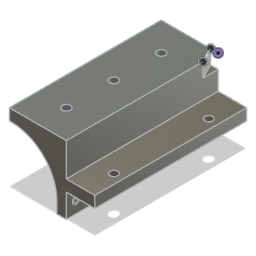
rear_mount_right_v2 (Autodesk Fusion 360 design; units mm, degrees)
Autodesk Fusion 360 part; units mm, degrees
note: some values were not read from the file. Set by a fixed rule: which sketch regions a step uses.
sketch "Esquisse1" plane through (0, 0, 0) normal (0, 0, 1) x (1, 0, 0)
  line L0 (15, 0) -> (0, 0)
  line L1 (0, 0) -> (0, 17.5)
  line L2 (0, 17.5) -> (-30, 17.5)
  line L3 (-30, 17.5) -> (-30, 11.5)
  line L4 (-30, 11.5) -> (-5, 11.5)
  line L5 (-5, 11.5) -> (-5, -18.5)
  line L6 (-5, -18.5) -> (0, -18.5)
  line L7 (0, -18.5) -> (0, -6)
  line L8 (0, -6) -> (15, -6)
  line L9 (15, -6) -> (15, 0)
  dimension "d1" = 12.5
  dimension "d2" = 6
  dimension "d3" = 5
  dimension "d4" = 15
  dimension "d6" = 6
  dimension "d7" = 30
  dimension "d46" = 36
  constraint coincident L0.end L1.start
  constraint horizontal L0
  constraint perpendicular L0 L1
  constraint perpendicular L1 L2
  constraint perpendicular L2 L3
  constraint perpendicular L3 L4
  constraint perpendicular L4 L5
  constraint perpendicular L5 L6
  constraint perpendicular L6 L7
  constraint perpendicular L7 L8
  constraint perpendicular L0 L9
  constraint collinear L1 L7
  measures "d1" distance of L6.end L7.end
  measures "d2" distance of L0.start L8.end
  measures "d3" distance of L5.end L6.end
  measures "d4" distance of L0.start L0.end
  measures "d6" distance of L2.end L3.end
  measures "d7" distance of L1 L3
  measures "d46" distance of L2 L6
extrude "Extrusion1" add sketch "Esquisse1" along normal blind 80
sketch "Esquisse2" plane through (0, -6, 0) normal (0, -1, 0) x (1, 0, 0)
  line L0 (0, 0) -> (15, 0)
  line L1 (15, 0) -> (15, 80)
  line L2 (15, 80) -> (0, 80)
  line L3 (0, 80) -> (0, 0)
  line L4 (10, 80) -> (10, 0) construction
  circle A0 centre (10, 65) radius 2.075
  circle A1 centre (10, 15) radius 2.075
  dimension "d10" = 4.15
  dimension "d11" = 15
  dimension "d12" = 15
  dimension "d38" = 10
  constraint coincident L4 A0.centre
  constraint coincident L4 A1.centre
  constraint equal A0 A1
  constraint vertical L4
  measures "d10" diameter of A1
  measures "d11" distance of L2 A0.centre
  measures "d12" distance of L0 A1.centre
  measures "d38" distance of L0.start L4
extrude "Extrusion2" cut sketch "Esquisse2" against normal blind 10 contours A0 | A1
sketch "Esquisse3" plane through (-5, 0, 0) normal (-1, 0, 0) x (0, 0, 1)
  line L0 (0, 11.5) -> (0, -18.5)
  line L1 (0, -18.5) -> (80, -18.5)
  line L2 (80, -18.5) -> (80, 11.5)
  line L3 (80, 11.5) -> (0, 11.5)
  line L4 (80, -12.25) -> (-7.1825, -12.25) construction
  circle A0 centre (19.5, -12.25) radius 1.75
  circle A1 centre (68, -12.25) radius 1.75
  circle A2 centre (75, -12.25) radius 1.75
  dimension "d15" = 6.25
  dimension "d16" = 3.5
  dimension "d17" = 5
  dimension "d18" = 7
  dimension "d19" = 60.5
  constraint coincident L2 L4.start
  constraint perpendicular L0 L4
  constraint coincident L4 A0.centre
  constraint coincident L4 A1.centre
  constraint coincident L4 A2.centre
  constraint equal A0 A1
  constraint equal A1 A2
  measures "d15" distance of L1 L4
  measures "d16" diameter of A0
  measures "d17" distance of L2 A2.centre
  measures "d18" distance of A1.centre A2.centre
  measures "d19" distance of L2 A0.centre
extrude "Extrusion3" cut sketch "Esquisse3" against normal blind 5 contours A0 | A1 | A2
fillet "Congé1" radius 24 1 edges at (-5, 11.5, 40)
sketch "Esquisse4" plane through (0, 17.5, 0) normal (0, 1, 0) x (-1, 0, 0)
  line L0 (0, 0) -> (30, 0)
  line L1 (30, 0) -> (30, 80)
  line L2 (30, 80) -> (0, 80)
  line L3 (0, 80) -> (0, 0)
  line L4 (15, 0) -> (15, 80) construction
  circle A0 centre (15, 15) radius 2.175
  circle A1 centre (15, 40) radius 2.175
  circle A2 centre (15, 65) radius 2.175
  dimension "d25" = 4.35
  dimension "d26" = 40
  dimension "d27" = 15
  dimension "d28" = 15
  dimension "d36" = 65
  dimension "d37" = 15
  dimension "d44" = 15
  constraint coincident L0 L4.start
  constraint perpendicular L2 L4
  constraint coincident L4 A0.centre
  constraint midpoint L4 A1.centre
  constraint coincident L4 A2.centre
  constraint equal A1 A2
  constraint equal A0 A1
  measures "d25" diameter of A2
  measures "d26" distance of L2 A1.centre
  measures "d27" distance of L2 A2.centre
  measures "d28" distance of L0 A0.centre
  measures "d36" distance of L4.end A0.centre
  measures "d37" distance of L2.end L4.end
  measures "d44" distance of L1.end L4.end
extrude "Extrusion4" cut sketch "Esquisse4" against normal blind 33 contours A0 | A1 | A2
sketch "Esquisse5" plane through (0, 17.5, 0) normal (0, 1, 0) x (-1, 0, 0)
  circle A0 centre (15, 15) radius 2.175
  circle A1 centre (15, 40) radius 2.175
  circle A2 centre (15, 65) radius 2.175
  line L0 (0, 0) -> (30, 0)
  line L1 (30, 0) -> (30, 80)
  line L2 (30, 80) -> (0, 80)
  line L3 (0, 80) -> (0, 0)
  line L4 (0, 8) -> (4, 0)
  dimension "d31" = 8
  dimension "d32" = 4
  constraint coincident L3 L4.start
  constraint coincident L0 L4.end
  measures "d31" distance of L0.start L4.start
  measures "d32" distance of L0.start L4.end
extrude "Extrusion5" cut sketch "Esquisse5" against normal blind 7.5 contours L0 L3 L4
sketch "Esquisse6" plane through (0, 11.5, 0) normal (0, -1, 0) x (1, 0, 0)
  line L0 (-29, 0) -> (-29, 80)
  line L1 (-29, 80) -> (-30, 80)
  line L2 (-30, 80) -> (-30, 0)
  line L3 (-30, 0) -> (-29, 0)
  circle A0 centre (-15, 15) radius 4
  circle A1 centre (-15, 40) radius 4
  circle A2 centre (-15, 65) radius 4
  dimension "d39" = 8
  constraint equal A1 A2
  constraint equal A0 A1
  measures "d39" diameter of A1
extrude "Extrusion6" cut sketch "Esquisse6" along normal blind 16 contours A0 | A1 | A2
sketch "Esquisse8" plane through (0, 12.5, 0) normal (0, -1, 0) x (1, 0, 0)
  circle A0 centre (-15, 65) radius 1.575
  circle A1 centre (-15, 65) radius 2.175
  circle A2 centre (-15, 65) radius 4
  circle A3 centre (-15, 14.9898) radius 4
  circle A4 centre (-15, 40) radius 4
  circle A5 centre (-15, 40) radius 2.175
  dimension "d45" = 8
  constraint concentric A0 A2
  constraint concentric A4 A5
  constraint equal A2 A4
  constraint equal A3 A4
  measures "d45" diameter of A3
equation "d12 = d11"
equation "d15 = ( 12.5 / 2 ) * 1 mm"
